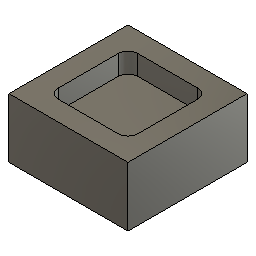
pocketing (Autodesk Fusion 360 design; units mm, degrees)
Autodesk Fusion 360 part; units mm, degrees
sketch "Sketch1" plane through (0, 0, 0) normal (0, 1, 0) x (1, 0, 0)
  line L0 (0, 0) -> (60, 0)
  line L1 (60, 0) -> (60, -60)
  line L2 (60, -60) -> (0, -60)
  line L3 (0, -60) -> (0, 0)
  dimension "d1" = 60
  dimension "d2" = 60
  constraint horizontal L0
  constraint vertical L1
  constraint horizontal L2
  constraint vertical L3
  constraint coincident L0.start L3.end
  measures "d1" distance of L0.start L0.end
  measures "d2" distance of L0.start L2.end
extrude "Extrude1" add sketch "Sketch1" along normal blind 50
sketch "Sketch2" plane through (0, 50, 0) normal (0, 1, 0) x (-1, 0, 0)
  line L0 (0, 60) -> (-60, 60)
  line L1 (-60, 60) -> (-60, 0)
  line L2 (-60, 0) -> (0, 0)
  line L3 (0, 0) -> (0, 60)
  line L4 (-10, 10) -> (-50, 10)
  line L5 (-50, 10) -> (-50, 50)
  line L6 (-50, 50) -> (-10, 50)
  line L7 (-10, 50) -> (-10, 10)
  dimension "d5" = 10
  dimension "d6" = 10
  dimension "d7" = 10
  dimension "d8" = 10
  constraint horizontal L4
  constraint vertical L5
  constraint horizontal L6
  constraint vertical L7
  measures "d5" distance of L3 L7
  measures "d6" distance of L1 L5
  measures "d7" distance of L0 L6
  measures "d8" distance of L2 L4
extrude "Extrude2" cut 1 faces at (20, 0, 20) along direction (0, 1, 0) blind 20
extrude "Extrude3" cut sketch "Sketch2" against normal blind 10 contours L4 L5 L6 L7
fillet "Fillet1" radius 5 4 edges at (10, 45, 10) (10, 45, 50) (50, 45, 50) (50, 45, 10)
